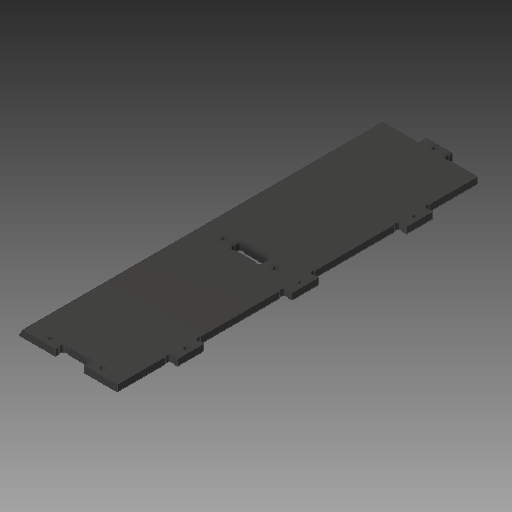
# Autodesk Inventor part: BA03
Saved by Autodesk Inventor 2017 (Build 210142000, 142)
## iProperties
Created: 2019-05-22
Part Number: BA03
Material: Polyethylene, High Density
Document SubType Name: Modeling
Designer: Dell
Density: 0.952 g/cm^3
Appearance: Smooth - Black
Mass: 197.865 g
Surface Area: 731.846 cm^2
Volume: 207.842 cm^3
Author: Dell
Autodesk Inventor part; units mm, degrees
ref_plane "YZ Plane" through (0, 0, 0) normal (1, 0, 0) x (0, 1, 0)
ref_plane "XZ Plane" through (0, 0, 0) normal (0, 1, 0) x (-1, 0, 0)
sketch "Sketch1" plane through (0, 0, 0) normal (0, 0, 1) x (1, 0, 0)
  line L0 (0, 0) -> (95.25, 0)
  line L1 (95.25, 0) -> (95.25, 6.35)
  line L2 (95.25, 6.35) -> (3.6662, 6.35)
  line L3 (3.6662, 6.35) -> (0, 0)
  dimension "d0" = 95.25
  dimension "d1" = 6.35
  dimension "d2" = 60
  constraints: 8 end point, 2 perpendicular, 1 horizontal
  measures "d0" distance of L0.start L0.end
  measures "d1" distance of L0.end L1.end
  measures "d2" angle of L0 L3
extrude "Extrusion1" add sketch "Sketch1" along normal blind 349.25
sketch "Sketch2" plane through (0, 0, 0) normal (0, -1, 0) x (1, 0, 0)
  line L0 (38.1, 349.25) -> (63.5, 349.25)
  line L1 (63.5, 349.25) -> (63.5, 355.6)
  line L2 (63.5, 355.6) -> (38.1, 355.6)
  line L3 (38.1, 355.6) -> (38.1, 349.25)
  line L4 (0, 349.25) -> (101.6, 349.25)
  line L5 (0, 349.25) -> (95.25, 349.25) projected
  point P0 (0, 0)
  point P1 (50.8, 349.25)
  dimension "d5" = 25.4
  dimension "d6" = 6.35
  dimension "d9" = 101.6
  constraints: 10 end point, 2 midpoint, 2 parallel, 1 collinear, 1 horizontal, 1 perpendicular
  measures "d5" distance of L2.end L1.end
  measures "d6" distance of L1.end L0.end
  measures "d9" distance of L4.start L4.end
extrude "Extrusion2" add sketch "Sketch2" against normal blind 6.35
sketch "Sketch3" plane through (0, 0, 0) normal (0, -1, 0) x (1, 0, 0)
  line L0 (63.5, 349.25) -> (63.5, 355.6) projected
  line L1 (63.5, 355.6) -> (38.1, 355.6) projected
  circle A0 centre (50.8, 352.425) radius 2.25
  point P0 (0, 0)
  point P1 (50.8, 355.6)
  point P2 (63.5, 352.425)
  dimension "d10" = 4.5
  constraints: 2 midpoint, 1 centre point, 1 horizontal alignment, 1 vertical alignment
  measures "d10" diameter of A0
extrude "Extrusion3" cut sketch "Sketch3" against normal through all
sketch "Sketch4" plane through (0, 0, 0) normal (0, -1, 0) x (1, 0, 0)
  line L0 (95.25, 0) -> (95.25, 349.25) projected
  line L1 (95.25, 50.8) -> (101.6, 50.8)
  line L2 (101.6, 50.8) -> (101.6, 76.2)
  line L3 (101.6, 76.2) -> (95.25, 76.2)
  line L4 (95.25, 76.2) -> (95.25, 50.8)
  line L5 (95.25, 298.45) -> (101.6, 298.45)
  line L6 (101.6, 298.45) -> (101.6, 273.05)
  line L7 (101.6, 273.05) -> (95.25, 273.05)
  line L8 (95.25, 273.05) -> (95.25, 298.45)
  line L9 (95.25, 187.325) -> (101.6, 187.325)
  line L10 (101.6, 187.325) -> (101.6, 161.925)
  line L11 (101.6, 161.925) -> (95.25, 161.925)
  line L12 (95.25, 161.925) -> (95.25, 187.325)
  circle A0 centre (98.425, 285.75) radius 2.25
  circle A1 centre (98.425, 174.625) radius 2.25
  circle A2 centre (98.425, 63.5) radius 2.25
  point P0 (0, 0)
  point P1 (95.25, 174.625)
  point P2 (98.425, 298.45)
  point P3 (98.425, 187.325)
  point P4 (98.425, 76.2)
  point P5 (101.6, 285.75)
  point P6 (101.6, 174.625)
  point P7 (101.6, 63.5)
  dimension "d13" = 6.35
  dimension "d14" = 25.4
  dimension "d15" = 6.35
  dimension "d16" = 25.4
  dimension "d17" = 6.35
  dimension "d18" = 25.4
  dimension "d19" = 50.8
  dimension "d20" = 50.8
  dimension "d21" = 4.5
  dimension "d22" = 4.5
  dimension "d23" = 4.5
  constraints: 24 end point, 8 midpoint, 6 parallel, 3 centre point, 3 horizontal, 3 horizontal alignment, 3 perpendicular, 3 point on line, 3 vertical alignment
  measures "d13" distance of L3.end L2.end
  measures "d14" distance of L2.end L1.end
  measures "d15" distance of L6.end L7.end
  measures "d16" distance of L5.end L6.end
  measures "d17" distance of L10.end L11.end
  measures "d18" distance of L9.end L10.end
  measures "d19" distance from line of L0.end L5
  measures "d20" distance from line of L0.start L1
  measures "d21" diameter of A0
  measures "d22" diameter of A1
  measures "d23" diameter of A2
extrude "Extrusion4" add sketch "Sketch4" against normal blind 6.35
sketch "Sketch9" plane through (95.25, 0, 298.45) normal (0, 0, 1) x (1, 0, 0)
  line L0 (-95.25, 0) -> (0, 0) projected
  line L1 (-95.25, 0) -> (-95.25, 6.35)
  line L2 (0, 6.35) -> (-91.5838, 6.35) projected
  line L3 (-95.25, 6.35) -> (-91.5838, 6.35)
  line L4 (-91.5838, 6.35) -> (-95.25, 0)
  line L5 (-91.5838, 6.35) -> (-95.25, 0) projected
  constraints: 6 end point, 1 horizontal, 1 vertical
extrude "Extrusion9" [suppressed]
sketch "Sketch10" plane through (95.25, 0, 187.325) normal (0, 0, 1) x (1, 0, 0)
  line L0 (-81.5677, 12.7) -> (-88.9, 0) projected
  line L1 (-81.5677, 12.7) -> (-88.9, 12.7) projected
  line L2 (-88.9, 12.7) -> (-88.9, 0) projected
  point P0 (-95.25, 0)
extrude "Extrusion10" [suppressed]
sketch "Sketch11" plane through (95.25, 0, 76.2) normal (0, 0, 1) x (1, 0, 0)
  line L0 (-81.5677, 12.7) -> (-88.9, 0) projected
  line L1 (-81.5677, 12.7) -> (-88.9, 12.7) projected
  line L2 (-88.9, 12.7) -> (-88.9, 0) projected
  point P0 (-95.25, 0)
extrude "Extrusion11" [suppressed]
ref_plane "Work Plane1" through (0, 0, 174.625) normal (0, 0, 1) x (1, 0, 0)
mirror "Mirror1" about plane through (0, 0, 174.625) normal (0, 0, 1) of "Extrusion1", "Extrusion2", "Extrusion3", "Extrusion4"
sketch "Sketch12" plane through (3.6662, 6.35, 349.25) normal (0, 1, 0) x (1, 0, 0)
  line L0 (59.8338, 0) -> (59.8338, -6.35) projected
  line L1 (59.8338, -6.35) -> (59.8338, 0) projected
  line L2 (59.8338, -6.35) -> (34.4338, -6.35) projected
  line L3 (34.4338, -6.35) -> (59.8338, -6.35) projected
  line L4 (34.4338, 0) -> (34.4338, -6.35) projected
  line L5 (59.8338, 0) -> (34.4338, 0)
  line L6 (91.5838, 0) -> (59.8338, 0) projected
  line L7 (34.4338, -6.35) -> (59.8338, -6.35)
  line L8 (59.8338, -6.35) -> (59.8338, 0)
  line L9 (59.8338, 0) -> (34.4338, 0)
  line L10 (34.4338, 0) -> (34.4338, -6.35)
  point P0 (-3.6662, 349.25)
  constraints: 10 end point, 2 horizontal, 2 parallel, 1 perpendicular
extrude "Extrusion12" cut sketch "Sketch12" along normal through all both and the other way through all
sketch "Sketch13" plane through (3.6662, 6.35, 349.25) normal (0, 1, 0) x (1, 0, 0)
  circle A0 centre (20.7919, 6.35) radius 2.25
  line L0 (91.5838, 0) -> (0, 0) projected
  circle A1 centre (70.7919, 6.35) radius 2.25
  line L1 (33.0919, 0) -> (58.4919, 0)
  line L2 (58.4919, 0) -> (58.4919, 6.35)
  line L3 (58.4919, 6.35) -> (33.0919, 6.35)
  line L4 (33.0919, 6.35) -> (33.0919, 0)
  line L5 (20.7919, 6.35) -> (70.7919, 6.35) construction
  point P0 (-3.6662, 349.25)
  point P1 (45.7919, 6.35)
  point P2 (45.7919, 0)
  point P3 (45.7919, 0)
  dimension "d44" = 4.5
  dimension "d45" = 6.35
  dimension "d46" = 4.5
  dimension "d47" = 25.4
  dimension "d48" = 6.35
  dimension "d49" = 50
  constraints: 10 end point, 5 midpoint, 2 centre point, 2 horizontal, 2 parallel, 1 perpendicular, 1 vertical alignment
  measures "d44" diameter of A0
  measures "d45" distance from line of L0 L5.start
  measures "d46" diameter of A1
  measures "d47" distance of L3.end L2.end
  measures "d48" distance of L2.end L1.end
  measures "d49" distance of L5.start L5.end
extrude "Extrusion13" cut sketch "Sketch13" against normal through all
sketch "Sketch14" plane through (95.25, 0, 50.8) normal (0, -1, 0) x (1, 0, 0)
  line L0 (6.35, 111.125) -> (6.35, 136.525) projected
  line L1 (-33.0919, 292.1) -> (-58.4919, 292.1) projected
  line L2 (-58.4919, 127.475) -> (-33.0919, 127.475)
  line L3 (-33.0919, 127.475) -> (-33.0919, 121.125)
  line L4 (-33.0919, 121.125) -> (-58.4919, 121.125)
  line L5 (-58.4919, 121.125) -> (-58.4919, 127.475)
  point P0 (-95.25, -50.8)
  dimension "d54" = 6.35
  dimension "d55" = 10
  constraints: 8 end point, 2 parallel, 2 vertical alignment, 1 horizontal, 1 perpendicular
  measures "d54" distance of L4.end L2.start
  measures "d55" distance from line of L0.start L4
extrude "Extrusion14" cut sketch "Sketch14" against normal through all
sketch "Sketch15" plane through (95.25, 0, 50.8) normal (0, -1, 0) x (1, 0, 0)
  circle A0 centre (-70.7919, 124.3) radius 2.25
  circle A1 centre (-20.7919, 124.3) radius 2.25
  circle A2 centre (-70.7919, 292.1) radius 2.25 projected
  circle A3 centre (-20.7919, 292.1) radius 2.25 projected
  line L0 (-33.0919, 127.475) -> (-33.0919, 121.125) projected
  point P0 (-95.25, -50.8)
  point P1 (-33.0919, 124.3)
  point P2 (-33.0919, 124.3)
  dimension "d56" = 4.5
  dimension "d57" = 4.5
  constraints: 2 centre point, 2 horizontal alignment, 2 midpoint, 2 vertical alignment
  measures "d56" diameter of A0
  measures "d57" diameter of A1
extrude "Extrusion15" cut sketch "Sketch15" against normal through all contours A0 | A1
sketch "Sketch16" plane through (95.25, 6.35, 298.45) normal (0, 1, 0) x (1, 0, 0)
  line L0 (-59.7619, 127.795) -> (-31.8219, 127.795)
  line L1 (-31.8219, 127.795) -> (-31.8219, 118.905)
  line L2 (-31.8219, 118.905) -> (-59.7619, 118.905)
  line L3 (-59.7619, 118.905) -> (-59.7619, 127.795)
  line L4 (-95.25, -50.8) -> (-58.4919, -50.8) projected
  line L5 (-59.7619, -50.8) -> (-31.8219, -50.8)
  line L6 (-31.8219, -50.8) -> (-31.8219, -43.18)
  line L7 (-31.8219, -43.18) -> (-59.7619, -43.18)
  line L8 (-59.7619, -43.18) -> (-59.7619, -50.8)
  line L9 (-33.0919, 120.175) -> (-58.4919, 120.175) projected
  line L10 (-58.4919, -44.45) -> (-33.0919, -44.45) projected
  line L11 (-58.4919, 120.175) -> (-58.4919, 126.525) projected
  circle A0 centre (-59.3951, 300.6951) radius 3.175
  circle A1 centre (-29.5049, 300.6951) radius 3.175
  circle A2 centre (2.2451, 249.8951) radius 3.175
  circle A3 centre (2.2451, 220.0049) radius 3.175
  circle A4 centre (2.2451, 138.7701) radius 3.175
  circle A5 centre (2.2451, 108.8799) radius 3.175
  circle A6 centre (2.2451, 27.6451) radius 3.175
  circle A7 centre (2.2451, -2.2451) radius 3.175
  line L12 (-59.3951, 300.6951) -> (-57.15, 298.45)
  line L13 (-57.15, 304.8) -> (-57.15, 298.45) projected
  line L14 (0, 247.65) -> (2.2451, 249.8951)
  line L15 (6.35, 247.65) -> (0, 247.65) projected
  point P0 (-95.25, 298.45)
  point P1 (-45.7919, 120.175)
  point P2 (-45.7919, 118.905)
  point P3 (-45.7919, -43.18)
  point P4 (-45.7919, -44.45)
  point P5 (-58.4919, 123.35)
  point P6 (-59.7619, 123.35)
  point P7 (0, 0)
  point P8 (0, 25.4)
  point P9 (0, 111.125)
  point P10 (0, 136.525)
  point P11 (0, 222.25)
  point P12 (-31.75, 298.45)
  dimension "d63" = 6.35
  dimension "d64" = 6.35
  dimension "d65" = 6.35
  dimension "d66" = 6.35
  dimension "d67" = 6.35
  dimension "d68" = 6.35
  dimension "d69" = 6.35
  dimension "d70" = 6.35
  dimension "d60" = 1.27
  dimension "d61" = 1.27
  dimension "d62" = 1.27
  dimension "d77" = 45
  dimension "d78" = 45
  constraints: 20 end point, 9 vertical alignment, 6 midpoint, 4 parallel, 3 coincident, 3 point on line, 2 horizontal, 2 horizontal alignment, 2 perpendicular, 24 other
  measures "d60" distance between parallel lines of L2 L9
  measures "d61" distance between parallel lines of L3 L11
  measures "d62" distance between parallel lines of L7 L10
  measures "d77" angle of L13 L12
  measures "d78" angle of L14 L15
extrude "Extrusion16" cut sketch "Sketch16" against normal through all
sketch "Sketch17" plane through (101.6, 6.35, 298.45) normal (0, 1, 0) x (1, 0, 0)
  line L0 (-63.5, 304.8) -> (-38.1, 304.8)
  line L1 (-38.1, 304.8) -> (-38.1, 306.07)
  line L2 (-38.1, 306.07) -> (-63.5, 306.07)
  line L3 (-63.5, 306.07) -> (-63.5, 304.8)
  line L4 (0, 247.65) -> (1.27, 247.65)
  line L5 (1.27, 247.65) -> (1.27, 222.25)
  line L6 (1.27, 222.25) -> (0, 222.25)
  line L7 (0, 222.25) -> (0, 247.65)
  line L8 (0, 136.525) -> (1.27, 136.525)
  line L9 (1.27, 136.525) -> (1.27, 111.125)
  line L10 (1.27, 111.125) -> (0, 111.125)
  line L11 (0, 111.125) -> (0, 136.525)
  line L12 (0, 25.4) -> (1.27, 25.4)
  line L13 (1.27, 25.4) -> (1.27, 0)
  line L14 (1.27, 0) -> (0, 0)
  line L15 (0, 0) -> (0, 25.4)
  point P0 (-101.6, 298.45)
  dimension "d73" = 1.27
  dimension "d74" = 1.27
  constraints: 32 end point, 8 parallel, 4 coincident, 4 horizontal, 4 perpendicular, 1 point on line, 1 vertical alignment
  measures "d73" distance between parallel lines of L2 L0
  measures "d74" distance of L4.start L4.end
extrude "Extrusion17" add sketch "Sketch17" against normal up to surface (6.35 mm away) from surface at 0
sketch "Sketch18" plane through (3.6662, 6.35, 349.25) normal (0, 1, 0) x (1, 0, 0)
  line L0 (59.7619, 7.62) -> (59.7619, 0) construction
  line L1 (91.5838, 0) -> (59.7619, 0) construction
  line L2 (91.5838, 46.3099) -> (91.5838, 0) construction
  arc A0 (96.074, 50.8) -> (91.5838, 46.3099) centre (93.8289, 48.5549) ccw construction
  line L3 (96.074, 50.8) -> (99.2038, 50.8) construction
  line L4 (99.2038, 76.2) -> (99.2038, 50.8) construction
  line L5 (96.074, 76.2) -> (99.2038, 76.2) construction
  arc A1 (91.5838, 80.6901) -> (96.074, 76.2) centre (93.8289, 78.4451) ccw construction
  line L6 (91.5838, 157.4349) -> (91.5838, 80.6901) construction
  arc A2 (96.074, 161.925) -> (91.5838, 157.4349) centre (93.8289, 159.6799) ccw construction
  line L7 (96.074, 161.925) -> (99.2038, 161.925) construction
  line L8 (99.2038, 187.325) -> (99.2038, 161.925) construction
  line L9 (96.074, 187.325) -> (99.2038, 187.325) construction
  arc A3 (91.5838, 191.8151) -> (96.074, 187.325) centre (93.8289, 189.5701) ccw construction
  line L10 (91.5838, 268.5599) -> (91.5838, 191.8151) construction
  arc A4 (96.074, 273.05) -> (91.5838, 268.5599) centre (93.8289, 270.8049) ccw construction
  line L11 (96.074, 273.05) -> (99.2038, 273.05) construction
  line L12 (99.2038, 298.45) -> (99.2038, 273.05) construction
  line L13 (96.074, 298.45) -> (99.2038, 298.45) construction
  arc A5 (91.5838, 302.9401) -> (96.074, 298.45) centre (93.8289, 300.6951) ccw construction
  line L14 (91.5838, 349.25) -> (91.5838, 302.9401) construction
  line L15 (91.5838, 349.25) -> (64.324, 349.25) construction
  arc A6 (59.8338, 353.7401) -> (64.324, 349.25) centre (62.0789, 351.4951) ccw construction
  line L16 (59.8338, 356.87) -> (59.8338, 353.7401) construction
  line L17 (34.4338, 356.87) -> (59.8338, 356.87) construction
  line L18 (34.4338, 353.7401) -> (34.4338, 356.87) construction
  arc A7 (29.9437, 349.25) -> (34.4338, 353.7401) centre (32.1888, 351.4951) ccw construction
  line L19 (29.9437, 349.25) -> (0, 349.25) construction
  line L20 (0, 349.25) -> (0, 0) construction
  line L21 (31.8219, 0) -> (0, 0) construction
  line L22 (31.8219, 0) -> (31.8219, 7.62) construction
  line L23 (31.8219, 7.62) -> (59.7619, 7.62) construction
  line L24 (31.8219, 169.705) -> (31.8219, 178.595) construction
  line L25 (31.8219, 178.595) -> (59.7619, 178.595) construction
  line L26 (59.7619, 178.595) -> (59.7619, 169.705) construction
  line L27 (59.7619, 169.705) -> (31.8219, 169.705) construction
  circle A8 centre (20.7919, 174.15) radius 2.25 construction
  circle A9 centre (70.7919, 174.15) radius 2.25 construction
  circle A10 centre (94.7588, 285.75) radius 2.25 construction
  circle A11 centre (94.7588, 63.5) radius 2.25 construction
  circle A12 centre (94.7588, 174.625) radius 2.25 construction
  circle A13 centre (47.1338, 352.425) radius 2.25 construction
  circle A14 centre (20.7919, 6.35) radius 2.25 construction
  circle A15 centre (70.7919, 6.35) radius 2.25 construction
  line L28 (62.0789, 351.4951) -> (93.8289, 351.4951) construction
  line L29 (93.8289, 351.4951) -> (93.8289, 300.6951) construction
  line L30 (93.8289, 300.6951) -> (101.4489, 300.6951) construction
  line L31 (101.4489, 300.6951) -> (101.4489, 270.8049) construction
  line L32 (101.4489, 270.8049) -> (93.8289, 270.8049) construction
  line L33 (93.8289, 270.8049) -> (93.8289, 189.5701) construction
  line L34 (93.8289, 189.5701) -> (101.4489, 189.5701) construction
  line L35 (101.4489, 189.5701) -> (101.4489, 159.6799) construction
  line L36 (101.4489, 159.6799) -> (93.8289, 159.6799) construction
  line L37 (93.8289, 159.6799) -> (93.8289, 78.4451) construction
  line L38 (93.8289, 78.4451) -> (101.4489, 78.4451) construction
  line L39 (101.4489, 78.4451) -> (101.4489, 48.5549) construction
  line L40 (101.4489, 48.5549) -> (93.8289, 48.5549) construction
  line L41 (93.8289, 48.5549) -> (93.8289, -2.2451) construction
  line L42 (93.8289, -2.2451) -> (57.5168, -2.2451) construction
  line L43 (57.5168, -2.2451) -> (57.5168, 5.3749) construction
  line L44 (57.5168, 5.3749) -> (34.067, 5.3749) construction
  line L45 (34.067, 5.3749) -> (34.067, -2.2451) construction
  line L46 (34.067, -2.2451) -> (-2.2451, -2.2451) construction
  line L47 (-2.2451, -2.2451) -> (-2.2451, 351.4951) construction
  line L48 (-2.2451, 351.4951) -> (32.1888, 351.4951) construction
  line L49 (32.1888, 351.4951) -> (32.1888, 359.1151) construction
  line L50 (32.1888, 359.1151) -> (62.0789, 359.1151) construction
  line L51 (62.0789, 359.1151) -> (62.0789, 351.4951) construction
  line L52 (31.8219, 0) -> (31.8219, 7.62) projected
  circle A16 centre (34.067, 5.3749) radius 3.175
  line L53 (31.8219, 7.62) -> (59.7619, 7.62) projected
  circle A17 centre (57.5168, 5.3749) radius 3.175
  line L54 (57.5168, 176.3499) -> (34.067, 176.3499) construction
  line L55 (34.067, 176.3499) -> (34.067, 171.9501) construction
  line L56 (34.067, 171.9501) -> (57.5168, 171.9501) construction
  line L57 (57.5168, 171.9501) -> (57.5168, 176.3499) construction
  circle A18 centre (57.5168, 176.3499) radius 3.175
  line L58 (59.7619, 178.595) -> (59.7619, 169.705) projected
  circle A19 centre (57.5168, 171.9501) radius 3.175
  line L59 (31.8219, 169.705) -> (31.8219, 178.595) projected
  circle A20 centre (34.067, 171.9501) radius 3.175
  circle A21 centre (34.067, 176.3499) radius 3.175
  point P0 (-3.6662, 349.25)
  dimension "d79" = 6.35
  dimension "d80" = 6.35
  constraints: 56 end point, 6 coincident, 44 other
extrude "Extrusion18" cut sketch "Sketch18" against normal through all
equation "\"d1\" = Panel_Thickness"
equation "\"d6\" = Panel_Thickness"
equation "\"d7\" = Panel_Thickness"
equation "\"d13\" = Panel_Thickness"
equation "\"d15\" = Panel_Thickness"
equation "\"d17\" = Panel_Thickness"
equation "\"d24\" = Panel_Thickness"
equation "\"d48\" = Panel_Thickness"
equation "\"d54\" = Panel_Thickness"
equation "\"d63\" = Tool_Dia"
equation "\"d64\" = d63"
equation "\"d65\" = d63"
equation "\"d66\" = d63"
equation "\"d67\" = d63"
equation "\"d68\" = d63"
equation "\"d69\" = d63"
equation "\"d70\" = d63"
equation "\"d60\" = Fit_Tolerance"
equation "\"d61\" = Fit_Tolerance"
equation "\"d62\" = Fit_Tolerance"
equation "\"d73\" = Fit_Tolerance"
equation "\"d74\" = d73"
equation "\"d79\" = Tool_Dia"
equation "\"d80\" = Tool_Dia"
equation "\"Panel_Thickness\" = 6.35"
equation "\"Fit_Tolerance\" = 1.27"
equation "\"Tool_Dia\" = 6.35"
body "Solid1"
